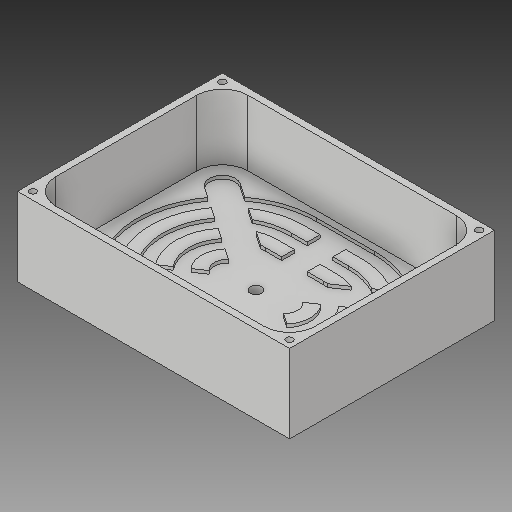
# Autodesk Inventor part: CorollaAirFilterCase
Saved by Autodesk Inventor 2018 (Build 220112000, 112)
## iProperties
Created: 2020-03-28
Part Number: CorollaAirFilterCase
Material: Generic
Document SubType Name: Modeling
Designer: emile
Density: 1 g/cm^3
Appearance: Default
Mass: 1009.29 g
Surface Area: 2532.41 cm^2
Volume: 1009.29 cm^3
Author: emile
Autodesk Inventor part; units mm, degrees
ref_plane "YZ Plane" through (0, 0, 0) normal (1, 0, 0) x (0, 1, 0)
ref_plane "XZ Plane" through (0, 0, 0) normal (0, 1, 0) x (-1, 0, 0)
ref_plane "XY Plane" through (0, 0, 0) normal (0, 0, 1) x (1, 0, 0)
sketch "Sketch1" plane through (0, 0, 0) normal (0, 1, 0) x (-1, 0, 0)
  line L0 (-128.5875, 95.25) -> (128.5875, 95.25)
  line L1 (128.5875, 95.25) -> (128.5875, -95.25)
  line L2 (128.5875, -95.25) -> (-128.5875, -95.25)
  line L3 (-128.5875, -95.25) -> (-128.5875, 95.25)
  line L4 (-128.5875, 95.25) -> (128.5875, -95.25) construction
  line L5 (128.5875, 95.25) -> (-128.5875, -95.25) construction
  line L6 (-115.8875, 82.55) -> (115.8875, 82.55)
  line L7 (115.8875, 82.55) -> (115.8875, -82.55)
  line L8 (115.8875, -82.55) -> (-115.8875, -82.55)
  line L9 (-115.8875, -82.55) -> (-115.8875, 82.55)
  line L10 (-115.8875, 82.55) -> (115.8875, -82.55) construction
  line L11 (115.8875, 82.55) -> (-115.8875, -82.55) construction
  line L12 (134.9375, -101.6) -> (134.9375, 101.6)
  line L13 (134.9375, 101.6) -> (-134.9375, 101.6)
  line L14 (-134.9375, 101.6) -> (-134.9375, -101.6)
  line L15 (-134.9375, -101.6) -> (134.9375, -101.6)
  point P0 (0, 0)
  point P1 (0, 0)
  dimension "d0" = 231.775
  dimension "d1" = 12.7
  dimension "d2" = 12.7
  dimension "d3" = 165.1
  dimension "d4" = 6.35
  constraints: 32 end point, 6 midpoint, 6 parallel, 3 perpendicular, 2 horizontal, 3 other
  measures "d0" distance between parallel lines of L9 L7
  measures "d1" distance between parallel lines of L1 L7
  measures "d2" distance between parallel lines of L2 L8
  measures "d3" distance of L6.end L7.end
  measures "d4" distance between parallel lines of L1 L12
extrude "Extrusion1" add sketch "Sketch1" along normal blind 65 contours L15 L14 L13 L12
extrude "Extrusion2" add sketch "Sketch1" against normal blind 12.7 contours L0 L1 L2 L3 | L6 L7 L8 L9 | L15 L14 L13 L12
fillet "Fillet1" radius 25.4 4 edges at (128.5875, 32.5, 95.25) (-128.5875, 32.5, 95.25) (-128.5875, 32.5, -95.25) (128.5875, 32.5, -95.25)
sketch "Sketch2" plane through (0, 0, 0) normal (0, 1, 0) x (1, 0, 0)
  line L0 (28.575, -88.9) -> (-28.575, -88.9)
  line L1 (-28.575, 88.9) -> (28.575, 88.9)
  arc A0 (28.575, -88.9) -> (28.575, 88.9) centre (28.575, 0) ccw
  arc A1 (-28.575, 88.9) -> (-28.575, -88.9) centre (-28.575, 0) ccw
  line L2 (28.575, 76.2) -> (-28.575, 76.2)
  arc A2 (-28.575, 76.2) -> (-28.575, -76.2) centre (-28.575, 0) ccw
  line L3 (-28.575, -76.2) -> (28.575, -76.2)
  arc A3 (28.575, -76.2) -> (28.575, 76.2) centre (28.575, 0) ccw
  line L4 (-28.575, 63.5) -> (28.575, 63.5)
  arc A4 (28.575, -63.5) -> (28.575, 63.5) centre (28.575, 0) ccw
  line L5 (28.575, -63.5) -> (-28.575, -63.5)
  arc A5 (-28.575, 63.5) -> (-28.575, -63.5) centre (-28.575, 0) ccw
  line L6 (28.575, 50.8) -> (-28.575, 50.8)
  arc A6 (-28.575, 50.8) -> (-28.575, -50.8) centre (-28.575, 0) ccw
  line L7 (-28.575, -50.8) -> (28.575, -50.8)
  arc A7 (28.575, -50.8) -> (28.575, 50.8) centre (28.575, 0) ccw
  line L8 (-28.575, 38.1) -> (28.575, 38.1)
  arc A8 (28.575, -38.1) -> (28.575, 38.1) centre (28.575, 0) ccw
  line L9 (28.575, -38.1) -> (-28.575, -38.1)
  arc A9 (-28.575, 38.1) -> (-28.575, -38.1) centre (-28.575, 0) ccw
  line L10 (28.575, 25.4) -> (-28.575, 25.4)
  arc A10 (-28.575, 25.4) -> (-28.575, -25.4) centre (-28.575, 0) ccw
  line L11 (-28.575, -25.4) -> (28.575, -25.4)
  arc A11 (28.575, -25.4) -> (28.575, 25.4) centre (28.575, 0) ccw
  line L12 (-28.575, 12.7) -> (28.575, 12.7)
  arc A12 (28.575, -12.7) -> (28.575, 12.7) centre (28.575, 0) ccw
  line L13 (28.575, -12.7) -> (-28.575, -12.7)
  arc A13 (-28.575, 12.7) -> (-28.575, -12.7) centre (-28.575, 0) ccw
  circle A14 centre (0, 0) radius 5.715
  point P0 (0, 12.7)
  dimension "d10" = 88.9
  dimension "d11" = 57.15
  dimension "d12" = 12.7
  dimension "d13" = 12.7
  dimension "d14" = 12.7
  dimension "d15" = 12.7
  dimension "d17" = 12.7
  dimension "d18" = 12.7
  dimension "d19" = 11.43
  constraints: 28 end point, 28 point on circle, 15 centre point, 7 parallel, 4 tangent, 2 horizontal alignment, 1 coincident, 1 midpoint, 1 vertical alignment, 18 other
  measures "d10" radius of A1
  measures "d11" distance of L1.start L1.end
  measures "d12" distance between parallel lines of L1 L2
  measures "d13" distance between parallel lines of L4 L2
  measures "d14" distance between parallel lines of L6 L4
  measures "d15" distance between parallel lines of L8 L10
  measures "d17" distance between parallel lines of L10 L12
  measures "d18" distance between parallel lines of L6 L8
  measures "d19" diameter of A14
extrude "Extrusion3" cut sketch "Sketch2" against normal through all contours A14
extrude "Extrusion4" cut sketch "Sketch2" against normal blind 3.175
sketch "Sketch3" plane through (0, 0, 0) normal (0, 1, 0) x (1, 0, 0)
  arc A0 (128.5875, 69.85) -> (103.1875, 95.25) centre (103.1875, 69.85) ccw projected
  line L0 (103.1875, 95.25) -> (-103.1875, 95.25) projected
  arc A1 (-103.1875, 95.25) -> (-128.5875, 69.85) centre (-103.1875, 69.85) ccw projected
  line L1 (-128.5875, 69.85) -> (-128.5875, -69.85) projected
  arc A2 (-128.5875, -69.85) -> (-103.1875, -95.25) centre (-103.1875, -69.85) ccw projected
  line L2 (-103.1875, -95.25) -> (103.1875, -95.25) projected
  arc A3 (103.1875, -95.25) -> (128.5875, -69.85) centre (103.1875, -69.85) ccw projected
  line L3 (128.5875, -69.85) -> (128.5875, 69.85) projected
  arc A4 (28.575, -88.9) -> (28.575, 88.9) centre (28.575, 0) ccw projected
  line L4 (28.575, -88.9) -> (-28.575, -88.9) projected
  arc A5 (-28.575, 88.9) -> (-28.575, -88.9) centre (-28.575, 0) ccw projected
  line L5 (-28.575, 88.9) -> (28.575, 88.9) projected
  line L6 (-12.7, -88.9) -> (12.7, -88.9)
  line L7 (12.7, -88.9) -> (12.7, 88.9)
  line L8 (12.7, 88.9) -> (-12.7, 88.9)
  line L9 (-12.7, 88.9) -> (-12.7, -88.9)
  line L10 (-12.7, -88.9) -> (12.7, 88.9) construction
  line L11 (12.7, -88.9) -> (-12.7, 88.9) construction
  line L12 (-28.575, 88.9) -> (28.575, 88.9) projected
  line L13 (103.1875, -69.85) -> (-103.1875, 69.85) construction
  circle A6 centre (0, 0) radius 5.715 projected
  line L14 (110.3067, -59.333) -> (-96.0683, 80.367)
  line L15 (-110.3067, 59.333) -> (96.0683, -80.367)
  arc A7 (96.0683, -80.367) -> (110.3067, -59.333) centre (103.1875, -69.85) ccw
  arc A8 (-96.0683, 80.367) -> (-110.3067, 59.333) centre (-103.1875, 69.85) ccw
  line L16 (-103.1875, -69.85) -> (103.1875, 69.85) construction
  line L17 (-96.0683, -80.367) -> (110.3067, 59.333)
  line L18 (96.0683, 80.367) -> (-110.3067, -59.333)
  arc A9 (-110.3067, -59.333) -> (-96.0683, -80.367) centre (-103.1875, -69.85) ccw
  arc A10 (110.3067, 59.333) -> (96.0683, 80.367) centre (103.1875, 69.85) ccw
  dimension "d24" = 25.4
  dimension "d25" = 25.4
  dimension "d26" = 25.4
  constraints: 28 end point, 8 point on circle, 8 tangent, 4 centre point, 4 midpoint, 4 parallel, 2 coincident, 1 horizontal, 1 perpendicular, 1 point on line
  measures "d24" distance between parallel lines of L9 L7
  measures "d25" distance between parallel lines of L18 L17
  measures "d26" distance between parallel lines of L15 L14
extrude "Extrusion5" cut sketch "Sketch3" against normal blind 3.175 contours L15 L7 L17 L14 A4 | A4 L14 A7 L15 | L4 L9 L17 L15 L7 | L15 L17 L7 | L17 L14 L7 L18 A4 | A4 L18 A10 L17 | L17 L7 L14 | L17 L15 L9 L18 L14 L7 | L17 L9 L15 | L17 A5 L18 L15 L9 | L14 L18 L7 | L15 L18 L9 | L17 A9 L18 A5 | L18 L14 L9 L5 L7 | L18 L9 L14 | L18 L15 A5 L14 L9 | L15 A8 L14 A5
sketch "Sketch4" plane through (0, 0, 0) normal (0, 1, 0) x (1, 0, 0)
  line L0 (-12.7, 23.9331) -> (-12.7, 25.4) projected
  line L1 (-12.7, 25.4) -> (-14.8671, 25.4) projected
  line L2 (-14.8671, 25.4) -> (-12.7, 23.9331) projected
  line L3 (12.7, 23.9331) -> (14.8671, 25.4) projected
  line L4 (14.8671, 25.4) -> (12.7, 25.4) projected
  line L5 (12.7, 25.4) -> (12.7, 23.9331) projected
  line L6 (12.7, -23.9331) -> (12.7, -25.4) projected
  line L7 (12.7, -25.4) -> (14.8671, -25.4) projected
  line L8 (14.8671, -25.4) -> (12.7, -23.9331) projected
  line L9 (-12.7, -25.4) -> (-12.7, -23.9331) projected
  line L10 (-12.7, -23.9331) -> (-14.8671, -25.4) projected
  line L11 (-14.8671, -25.4) -> (-12.7, -25.4) projected
  point P0 (0, 0)
extrude "Extrusion6" cut sketch "Sketch4" against normal blind 3.175
sketch "Sketch5" plane through (0, -12.7, 0) normal (0, -1, 0) x (1, 0, 0)
  point P0 (127.3175, 93.98)
  point P1 (-127.3175, 93.98)
  point P2 (-127.3175, -93.98)
  point P3 (127.3175, -93.98)
hole "Hole1" at (127.3175, -12.7, 93.98) at (-127.3175, -12.7, 93.98) at (-127.3175, -12.7, -93.98) at (127.3175, -12.7, -93.98) direction (0, 1, 0) diameter 6.7564 depth 77.7
equation "\"d2\" = d1"
equation "\"d13\" = d12"
equation "\"d14\" = d13"
equation "\"d15\" = d14"
equation "\"d17\" = d15"
equation "\"d18\" = d12"
equation "\"d25\" = d24"
equation "\"d26\" = d25"
body "Solid1"
